Autodesk Fusion 360 part; units mm, degrees
(part 3 of 4)
  line L296 (28.3401, 40.7282) -> (28.1058, 40.494)
  line L297 (25.2342, 40.494) -> (25, 40.7282)
  line L298 (28.1058, 40.494) -> (27.7742, 40.494)
  line L299 (28.1058, 40.494) -> (27.7742, 40.494)
  line L300 (25.8, 40.7282) -> (25.5658, 40.494)
  line L301 (28.3401, 41.0598) -> (28.3401, 40.7282)
  line L302 (25.8, 41.0598) -> (25.8, 40.7282)
  line L303 (25.5658, 41.294) -> (25.8, 41.0598)
  line L304 (25.5658, 40.494) -> (25.2342, 40.494)
  line L305 (25.2342, 41.294) -> (25.5658, 41.294)
  line L306 (25.2342, 41.294) -> (25.5658, 41.294)
  line L307 (25, 40.7282) -> (25, 41.0598)
  line L308 (25, 40.7282) -> (25, 41.0598)
  line L309 (25.8, 41.0598) -> (25.8, 40.7282)
  line L310 (25.5658, 41.294) -> (25.8, 41.0598)
  line L311 (25.8, 40.7282) -> (25.5658, 40.494)
  line L312 (25, 40.7282) -> (25, 41.0598)
  line L313 (25.5658, 40.494) -> (25.2342, 40.494)
  line L314 (25.2342, 45.2311) -> (25.5658, 45.2311)
  line L315 (28.1058, 45.2311) -> (28.3401, 44.9968)
  line L316 (28.1058, 45.2311) -> (28.3401, 44.9968)
  line L317 (28.3401, 44.6652) -> (28.1058, 44.431)
  line L318 (27.54, 44.6652) -> (27.54, 44.9968)
  line L319 (28.1058, 41.294) -> (28.3401, 41.0598)
  line L320 (25, 44.6652) -> (25, 44.9968)
  line L321 (27.7742, 45.2311) -> (28.1058, 45.2311)
  line L322 (28.3401, 44.9968) -> (28.3401, 44.6652)
  line L323 (28.3401, 41.0598) -> (28.3401, 40.7282)
  line L324 (27.54, 44.6652) -> (27.54, 44.9968)
  line L325 (27.54, 44.6652) -> (27.54, 44.9968)
  line L326 (25.8, 44.9968) -> (25.8, 44.6652)
  line L327 (27.54, 41.0598) -> (27.7742, 41.294)
  line L328 (25.5658, 45.2311) -> (25.8, 44.9968)
  line L329 (25.2342, 44.431) -> (25, 44.6652)
  line L330 (25.2342, 44.431) -> (25, 44.6652)
  line L331 (28.1058, 44.431) -> (27.7742, 44.431)
  line L332 (25.5658, 44.431) -> (25.2342, 44.431)
  line L333 (25, 44.6652) -> (25, 44.9968)
  line L334 (27.7742, 41.294) -> (28.1058, 41.294)
  line L335 (25.8, 44.6652) -> (25.5658, 44.431)
  line L336 (27.7742, 44.431) -> (27.54, 44.6652)
  line L337 (27.54, 40.7282) -> (27.54, 41.0598)
  line L338 (25.8, 44.6652) -> (25.5658, 44.431)
  line L339 (25, 44.6652) -> (25, 44.9968)
  line L340 (27.54, 44.9968) -> (27.7742, 45.2311)
  line L341 (28.3401, 44.6652) -> (28.1058, 44.431)
  line L342 (27.7742, 40.494) -> (27.54, 40.7282)
  line L343 (25, 44.9968) -> (25.2342, 45.2311)
  line L344 (10.1791, 41.1868) -> (10.1791, 40.8552)
  line L345 (9.3789, 41.1868) -> (9.6132, 41.4211)
  line L346 (25, 44.6652) -> (25, 44.9968)
  line L347 (12.1532, 40.621) -> (11.919, 40.8552)
  line L348 (9.6132, 41.4211) -> (9.9448, 41.4211)
  line L349 (12.7191, 41.1868) -> (12.7191, 40.8552)
  line L350 (25.5658, 44.431) -> (25.2342, 44.431)
  line L351 (10.1791, 40.8552) -> (9.9448, 40.621)
  line L352 (9.6132, 40.621) -> (9.3789, 40.8552)
  line L353 (27.7742, 45.2311) -> (28.1058, 45.2311)
  line L354 (28.1058, 44.431) -> (27.7742, 44.431)
  line L355 (27.54, 44.9968) -> (27.7742, 45.2311)
  line L356 (27.54, 44.6652) -> (27.54, 44.9968)
  line L357 (28.3401, 44.9968) -> (28.3401, 44.6652)
  line L358 (27.7742, 44.431) -> (27.54, 44.6652)
  line L359 (12.1532, 41.4211) -> (12.4848, 41.4211)
  line L360 (9.3789, 40.8552) -> (9.379, 41.1868)
  line L361 (12.7191, 41.1868) -> (12.7191, 40.8552)
  line L362 (11.919, 41.1868) -> (12.1532, 41.4211)
  line L363 (25.8, 44.9968) -> (25.8, 44.6652)
  line L364 (25.2342, 45.2311) -> (25.5658, 45.2311)
  line L365 (11.919, 40.8552) -> (11.919, 41.1868)
  line L366 (25, 44.9968) -> (25.2342, 45.2311)
  line L367 (12.7191, 40.8552) -> (12.4848, 40.621)
  line L368 (9.9448, 40.621) -> (9.6132, 40.621)
  line L369 (12.7191, 40.8552) -> (12.4848, 40.621)
  line L370 (25.5658, 45.2311) -> (25.8, 44.9968)
  line L371 (12.4848, 41.4211) -> (12.7191, 41.1868)
  arc A1067 (11.811, 48.133) -> (11.811, 48.895) centre (11.811, 48.514) ccw
  line L372 (11.811, 45.974) -> (10.287, 45.974)
  line L373 (10.414, 18.415) -> (8.89, 18.415)
  line L374 (9.6132, 41.4211) -> (9.9448, 41.4211)
  line L375 (17.554, 43.934) -> (16.046, 43.934)
  line L376 (11.811, 48.514) -> (10.287, 48.514)
  line L377 (10.414, 13.335) -> (8.89, 13.335)
  arc A1068 (10.414, 15.494) -> (10.414, 16.256) centre (10.414, 15.875) ccw
  line L378 (11.811, 45.974) -> (10.287, 45.974)
  line L379 (12.4848, 40.621) -> (12.1532, 40.621)
  line L380 (10.1791, 41.1868) -> (10.1791, 40.8552)
  arc A1069 (10.287, 48.895) -> (10.287, 48.133) centre (10.287, 48.514) ccw
  line L381 (11.811, 48.514) -> (10.287, 48.514)
  arc A1070 (10.287, 46.355) -> (10.287, 45.593) centre (10.287, 45.974) ccw
  line L382 (9.6132, 40.621) -> (9.3789, 40.8552)
  arc A1071 (10.287, 46.355) -> (10.287, 45.593) centre (10.287, 45.974) ccw
  line L383 (12.7191, 41.1868) -> (12.7191, 40.8552)
  line L384 (9.3789, 40.8552) -> (9.379, 41.1868)
  line L385 (11.919, 40.8552) -> (11.919, 41.1868)
  line L386 (12.4848, 41.4211) -> (12.7191, 41.1868)
  arc A1072 (11.811, 45.593) -> (11.811, 46.355) centre (11.811, 45.974) ccw
  line L387 (17.554, 42.426) -> (17.554, 43.934)
  line L388 (10.414, 15.875) -> (8.89, 15.875)
  line L389 (9.9448, 40.621) -> (9.6132, 40.621)
  arc A1073 (8.89, 18.796) -> (8.89, 18.034) centre (8.89, 18.415) ccw
  line L390 (9.3789, 41.1868) -> (9.6132, 41.4211)
  arc A1074 (11.811, 48.133) -> (11.811, 48.895) centre (11.811, 48.514) ccw
  line L391 (10.414, 13.335) -> (8.89, 13.335)
  line L392 (12.4848, 40.621) -> (12.1532, 40.621)
  arc A1075 (10.414, 18.034) -> (10.414, 18.796) centre (10.414, 18.415) ccw
  arc A1076 (8.89, 16.256) -> (8.89, 15.494) centre (8.89, 15.875) ccw
  arc A1077 (10.287, 48.895) -> (10.287, 48.133) centre (10.287, 48.514) ccw
  arc A1078 (8.89, 18.796) -> (8.89, 18.034) centre (8.89, 18.415) ccw
  line L393 (10.1791, 41.1868) -> (10.1791, 40.8552)
  line L394 (12.1532, 40.621) -> (11.919, 40.8552)
  line L395 (9.9448, 41.4211) -> (10.1791, 41.1868)
  line L396 (10.1791, 41.1868) -> (10.1791, 40.8552)
  line L397 (10.414, 18.415) -> (8.89, 18.415)
  line L398 (16.046, 42.426) -> (17.554, 42.426)
  line L399 (11.919, 41.1868) -> (12.1532, 41.4211)
  line L400 (12.7191, 41.1868) -> (12.7191, 40.8552)
  line L401 (9.9448, 41.4211) -> (10.1791, 41.1868)
  line L402 (12.1532, 41.4211) -> (12.4848, 41.4211)
  line L403 (10.1791, 40.8552) -> (9.9448, 40.621)
  arc A1079 (11.811, 45.593) -> (11.811, 46.355) centre (11.811, 45.974) ccw
  arc A1080 (10.414, 18.034) -> (10.414, 18.796) centre (10.414, 18.415) ccw
  line L404 (23.7998, 7.7568) -> (23.9932, 7.9502)
  line L405 (24.4602, 15.1032) -> (24.2668, 14.9098)
  line L406 (24.4602, 7.7568) -> (24.4602, 7.4832)
  line L407 (24.4602, 15.1032) -> (24.2668, 14.9098)
  line L408 (23.9932, 14.9098) -> (23.7998, 15.1032)
  line L409 (24.2668, 7.2898) -> (23.9932, 7.2898)
  line L410 (24.2668, 14.9098) -> (23.9932, 14.9098)
  line L411 (24.4602, 7.7568) -> (24.4602, 7.4832)
  line L412 (23.9932, 15.5702) -> (24.2668, 15.5702)
  line L413 (24.2668, 14.9098) -> (23.9932, 14.9098)
  line L414 (24.2668, 15.5702) -> (24.4602, 15.3768)
  line L415 (24.2668, 14.9098) -> (23.9932, 14.9098)
  line L416 (23.9932, 15.5702) -> (24.2668, 15.5702)
  line L417 (24.2668, 7.2898) -> (23.9932, 7.2898)
  arc A1081 (10.414, 15.494) -> (10.414, 16.256) centre (10.414, 15.875) ccw
  arc A1082 (16.423, 48.26) -> (17.177, 48.26) centre (16.8, 48.26) ccw
  line L418 (24.4602, 7.4832) -> (24.2668, 7.2898)
  line L419 (24.2668, 7.2898) -> (23.9932, 7.2898)
  line L420 (23.9932, 14.9098) -> (23.7998, 15.1032)
  line L421 (24.4602, 15.3768) -> (24.4602, 15.1032)
  line L422 (24.2668, 7.2898) -> (23.9932, 7.2898)
  arc A1083 (17.177, 48.26) -> (16.423, 48.26) centre (16.8, 48.26) ccw
  line L423 (24.2668, 7.9502) -> (24.4602, 7.7568)
  line L424 (23.7998, 15.1032) -> (23.7998, 15.3768)
  arc A1084 (10.414, 12.954) -> (10.414, 13.716) centre (10.414, 13.335) ccw
  line L425 (10.414, 15.875) -> (8.89, 15.875)
  line L426 (17.554, 43.934) -> (16.046, 43.934)
  arc A1085 (16.423, 45.72) -> (17.177, 45.72) centre (16.8, 45.72) ccw
  line L427 (16.046, 42.426) -> (17.554, 42.426)
  line L428 (23.9932, 7.9502) -> (24.2668, 7.9502)
  arc A1086 (17.177, 45.72) -> (16.423, 45.72) centre (16.8, 45.72) ccw
  arc A1087 (8.89, 13.716) -> (8.89, 12.954) centre (8.89, 13.335) ccw
  arc A1088 (17.177, 48.26) -> (16.423, 48.26) centre (16.8, 48.26) ccw
  line L429 (24.2668, 15.5702) -> (24.4602, 15.3768)
  line L430 (23.7998, 7.7568) -> (23.9932, 7.9502)
  line L431 (23.7998, 15.3768) -> (23.9932, 15.5702)
  line L432 (16.046, 43.934) -> (16.046, 42.426)
  line L433 (23.7998, 15.1032) -> (23.7998, 15.3768)
  arc A1089 (27.686, 29.21) -> (27.686, 29.972) centre (27.686, 29.591) ccw
  line L434 (27.686, 34.671) -> (26.162, 34.671)
  arc A1090 (8.89, 13.716) -> (8.89, 12.954) centre (8.89, 13.335) ccw
  line L435 (24.4602, 7.4832) -> (24.2668, 7.2898)
  arc A1091 (26.162, 27.432) -> (26.162, 26.67) centre (26.162, 27.051) ccw
  line L436 (24.2668, 14.9098) -> (23.9932, 14.9098)
  line L437 (27.686, 32.131) -> (26.162, 32.131)
  arc A1092 (16.423, 48.26) -> (17.177, 48.26) centre (16.8, 48.26) ccw
  arc A1093 (17.177, 45.72) -> (16.423, 45.72) centre (16.8, 45.72) ccw
  line L438 (24.2668, 7.9502) -> (24.4602, 7.7568)
  line L439 (23.9932, 7.9502) -> (24.2668, 7.9502)
  line L440 (16.046, 43.934) -> (16.046, 42.426)
  line L441 (23.9932, 7.2898) -> (23.7998, 7.4832)
  arc A1094 (16.423, 45.72) -> (17.177, 45.72) centre (16.8, 45.72) ccw
  arc A1095 (8.89, 16.256) -> (8.89, 15.494) centre (8.89, 15.875) ccw
  line L442 (17.554, 42.426) -> (17.554, 43.934)
  line L443 (23.7998, 7.4832) -> (23.7998, 7.7568)
  arc A1096 (10.414, 12.954) -> (10.414, 13.716) centre (10.414, 13.335) ccw
  line L444 (23.7998, 7.4832) -> (23.7998, 7.7568)
  line L445 (23.9932, 7.2898) -> (23.7998, 7.4832)
  line L446 (24.4602, 15.3768) -> (24.4602, 15.1032)
  line L447 (23.7998, 15.3768) -> (23.9932, 15.5702)
  arc A1097 (27.686, 36.83) -> (27.686, 37.592) centre (27.686, 37.211) ccw
  line L448 (27.686, 34.671) -> (26.162, 34.671)
  arc A1098 (26.162, 32.512) -> (26.162, 31.75) centre (26.162, 32.131) ccw
  arc A1099 (27.686, 31.75) -> (27.686, 32.512) centre (27.686, 32.131) ccw
  arc A1100 (27.686, 34.29) -> (27.686, 35.052) centre (27.686, 34.671) ccw
  arc A1101 (27.686, 36.83) -> (27.686, 37.592) centre (27.686, 37.211) ccw
  arc A1102 (26.162, 35.052) -> (26.162, 34.29) centre (26.162, 34.671) ccw
  line L449 (27.686, 37.211) -> (26.162, 37.211)
  line L450 (27.686, 29.591) -> (26.162, 29.591)
  arc A1103 (26.162, 29.972) -> (26.162, 29.21) centre (26.162, 29.591) ccw
  line L451 (27.686, 19.431) -> (26.162, 19.431)
  line L452 (27.686, 27.051) -> (26.162, 27.051)
  arc A1104 (27.686, 26.67) -> (27.686, 27.432) centre (27.686, 27.051) ccw
  arc A1105 (26.162, 24.892) -> (26.162, 24.13) centre (26.162, 24.511) ccw
  arc A1106 (27.686, 24.13) -> (27.686, 24.892) centre (27.686, 24.511) ccw
  line L453 (27.686, 19.431) -> (26.162, 19.431)
  arc A1107 (26.162, 19.812) -> (26.162, 19.05) centre (26.162, 19.431) ccw
  line L454 (27.686, 21.971) -> (26.162, 21.971)
  arc A1108 (27.686, 34.29) -> (27.686, 35.052) centre (27.686, 34.671) ccw
  line L455 (27.686, 24.511) -> (26.162, 24.511)
  arc A1109 (26.162, 22.352) -> (26.162, 21.59) centre (26.162, 21.971) ccw
  arc A1110 (27.686, 24.13) -> (27.686, 24.892) centre (27.686, 24.511) ccw
  arc A1111 (26.162, 27.432) -> (26.162, 26.67) centre (26.162, 27.051) ccw
  arc A1112 (27.686, 19.05) -> (27.686, 19.812) centre (27.686, 19.431) ccw
  arc A1113 (27.686, 26.67) -> (27.686, 27.432) centre (27.686, 27.051) ccw
  arc A1114 (26.162, 22.352) -> (26.162, 21.59) centre (26.162, 21.971) ccw
  line L456 (27.686, 21.971) -> (26.162, 21.971)
  line L457 (27.686, 29.591) -> (26.162, 29.591)
  line L458 (27.686, 27.051) -> (26.162, 27.051)
  line L459 (27.686, 32.131) -> (26.162, 32.131)
  line L460 (27.686, 24.511) -> (26.162, 24.511)
  arc A1115 (27.686, 21.59) -> (27.686, 22.352) centre (27.686, 21.971) ccw
  arc A1116 (27.686, 29.21) -> (27.686, 29.972) centre (27.686, 29.591) ccw
  arc A1117 (26.162, 37.592) -> (26.162, 36.83) centre (26.162, 37.211) ccw
  arc A1118 (26.162, 35.052) -> (26.162, 34.29) centre (26.162, 34.671) ccw
  line L461 (27.686, 37.211) -> (26.162, 37.211)
  arc A1119 (27.686, 21.59) -> (27.686, 22.352) centre (27.686, 21.971) ccw
  arc A1120 (26.162, 32.512) -> (26.162, 31.75) centre (26.162, 32.131) ccw
  arc A1121 (13.462, 19.812) -> (13.462, 19.05) centre (13.462, 19.431) ccw
  arc A1122 (13.462, 32.512) -> (13.462, 31.75) centre (13.462, 32.131) ccw
  arc A1123 (13.462, 22.352) -> (13.462, 21.59) centre (13.462, 21.971) ccw
  arc A1124 (27.686, 19.05) -> (27.686, 19.812) centre (27.686, 19.431) ccw
  arc A1125 (26.162, 24.892) -> (26.162, 24.13) centre (26.162, 24.511) ccw
  arc A1126 (26.162, 37.592) -> (26.162, 36.83) centre (26.162, 37.211) ccw
  arc A1127 (27.686, 31.75) -> (27.686, 32.512) centre (27.686, 32.131) ccw
  line L462 (13.462, 24.511) -> (14.986, 24.511)
  arc A1128 (13.462, 22.352) -> (13.462, 21.59) centre (13.462, 21.971) ccw
  arc A1129 (13.462, 24.892) -> (13.462, 24.13) centre (13.462, 24.511) ccw
  arc A1130 (14.986, 29.21) -> (14.986, 29.972) centre (14.986, 29.591) ccw
  line L463 (13.462, 19.431) -> (14.986, 19.431)
  arc A1131 (14.986, 19.05) -> (14.986, 19.812) centre (14.986, 19.431) ccw
  arc A1132 (26.162, 19.812) -> (26.162, 19.05) centre (26.162, 19.431) ccw
  line L464 (13.462, 24.511) -> (14.986, 24.511)
  arc A1133 (13.462, 29.972) -> (13.462, 29.21) centre (13.462, 29.591) ccw
  arc A1134 (26.162, 29.972) -> (26.162, 29.21) centre (26.162, 29.591) ccw
  arc A1135 (14.986, 19.05) -> (14.986, 19.812) centre (14.986, 19.431) ccw
  line L465 (13.462, 21.971) -> (14.986, 21.971)
  arc A1136 (14.986, 31.75) -> (14.986, 32.512) centre (14.986, 32.131) ccw
  arc A1137 (14.986, 29.21) -> (14.986, 29.972) centre (14.986, 29.591) ccw
  arc A1138 (13.462, 27.432) -> (13.462, 26.67) centre (13.462, 27.051) ccw
  line L466 (13.462, 29.591) -> (14.986, 29.591)
  line L467 (13.462, 32.131) -> (14.986, 32.131)
  line L468 (13.462, 37.211) -> (14.986, 37.211)
  line L469 (13.462, 27.051) -> (14.986, 27.051)
  arc A1139 (14.986, 26.67) -> (14.986, 27.432) centre (14.986, 27.051) ccw
  arc A1140 (14.986, 21.59) -> (14.986, 22.352) centre (14.986, 21.971) ccw
  arc A1141 (14.986, 24.13) -> (14.986, 24.892) centre (14.986, 24.511) ccw
  arc A1142 (13.462, 32.512) -> (13.462, 31.75) centre (13.462, 32.131) ccw
  arc A1143 (13.462, 29.972) -> (13.462, 29.21) centre (13.462, 29.591) ccw
  line L470 (13.462, 34.671) -> (14.986, 34.671)
  line L471 (13.462, 29.591) -> (14.986, 29.591)
  arc A1144 (13.462, 35.052) -> (13.462, 34.29) centre (13.462, 34.671) ccw
  line L472 (13.462, 32.131) -> (14.986, 32.131)
  arc A1145 (13.462, 35.052) -> (13.462, 34.29) centre (13.462, 34.671) ccw
  line L473 (13.462, 34.671) -> (14.986, 34.671)
  arc A1146 (14.986, 34.29) -> (14.986, 35.052) centre (14.986, 34.671) ccw
  arc A1147 (13.462, 27.432) -> (13.462, 26.67) centre (13.462, 27.051) ccw
  arc A1148 (14.986, 34.29) -> (14.986, 35.052) centre (14.986, 34.671) ccw
  line L474 (13.462, 21.971) -> (14.986, 21.971)
  arc A1149 (30.8896, 34.935) -> (29.9244, 34.935) centre (30.407, 34.935) ccw
  line L475 (13.462, 37.211) -> (14.986, 37.211)
  arc A1150 (14.986, 36.83) -> (14.986, 37.592) centre (14.986, 37.211) ccw
  arc A1151 (5.4846, 24.775) -> (4.5194, 24.775) centre (5.002, 24.775) ccw
  arc A1152 (4.5194, 34.935) -> (5.4846, 34.935) centre (5.002, 34.935) ccw
  arc A1153 (4.5194, 42.555) -> (5.4846, 42.555) centre (5.002, 42.555) ccw
  arc A1154 (14.986, 36.83) -> (14.986, 37.592) centre (14.986, 37.211) ccw
  arc A1155 (13.462, 37.592) -> (13.462, 36.83) centre (13.462, 37.211) ccw
  arc A1156 (14.986, 26.67) -> (14.986, 27.432) centre (14.986, 27.051) ccw
  arc A1157 (5.4846, 14.615) -> (4.5194, 14.615) centre (5.002, 14.615) ccw
  arc A1158 (4.5194, 42.555) -> (5.4846, 42.555) centre (5.002, 42.555) ccw
  arc A1159 (4.5194, 24.775) -> (5.4846, 24.775) centre (5.002, 24.775) ccw
  arc A1160 (5.4846, 42.555) -> (4.5194, 42.555) centre (5.002, 42.555) ccw
  arc A1161 (4.5194, 14.615) -> (5.4846, 14.615) centre (5.002, 14.615) ccw
  arc A1162 (13.462, 24.892) -> (13.462, 24.13) centre (13.462, 24.511) ccw
  line L476 (13.462, 19.431) -> (14.986, 19.431)
  arc A1163 (14.986, 31.75) -> (14.986, 32.512) centre (14.986, 32.131) ccw
  arc A1164 (14.986, 21.59) -> (14.986, 22.352) centre (14.986, 21.971) ccw
  arc A1165 (29.9244, 34.935) -> (30.8896, 34.935) centre (30.407, 34.935) ccw
  arc A1166 (14.986, 24.13) -> (14.986, 24.892) centre (14.986, 24.511) ccw
  line L477 (13.462, 27.051) -> (14.986, 27.051)
  arc A1167 (13.462, 19.812) -> (13.462, 19.05) centre (13.462, 19.431) ccw
  arc A1168 (13.462, 37.592) -> (13.462, 36.83) centre (13.462, 37.211) ccw
  arc A1169 (4.5194, 12.075) -> (5.4846, 12.075) centre (5.002, 12.075) ccw
  arc A1170 (5.4846, 34.935) -> (4.5194, 34.935) centre (5.002, 34.935) ccw
  arc A1171 (5.4846, 14.615) -> (4.5194, 14.615) centre (5.002, 14.615) ccw
  arc A1172 (4.5194, 32.395) -> (5.4846, 32.395) centre (5.002, 32.395) ccw
  arc A1173 (5.4846, 34.935) -> (4.5194, 34.935) centre (5.002, 34.935) ccw
  arc A1174 (4.5194, 32.395) -> (5.4846, 32.395) centre (5.002, 32.395) ccw
  arc A1175 (5.4846, 32.395) -> (4.5194, 32.395) centre (5.002, 32.395) ccw
  arc A1176 (5.4846, 24.775) -> (4.5194, 24.775) centre (5.002, 24.775) ccw
  arc A1177 (5.4846, 12.075) -> (4.5194, 12.075) centre (5.002, 12.075) ccw
  arc A1178 (4.5194, 12.075) -> (5.4846, 12.075) centre (5.002, 12.075) ccw
  arc A1179 (4.5194, 14.615) -> (5.4846, 14.615) centre (5.002, 14.615) ccw
  arc A1180 (5.4846, 32.395) -> (4.5194, 32.395) centre (5.002, 32.395) ccw
  arc A1181 (5.4846, 12.075) -> (4.5194, 12.075) centre (5.002, 12.075) ccw
  arc A1182 (4.5194, 34.935) -> (5.4846, 34.935) centre (5.002, 34.935) ccw
  arc A1183 (5.4846, 42.555) -> (4.5194, 42.555) centre (5.002, 42.555) ccw
  arc A1184 (4.5194, 19.695) -> (5.4846, 19.695) centre (5.002, 19.695) ccw
  arc A1185 (29.9244, 32.395) -> (30.8896, 32.395) centre (30.407, 32.395) ccw
  arc A1186 (29.9244, 24.775) -> (30.8896, 24.775) centre (30.407, 24.775) ccw
  arc A1187 (29.9244, 34.935) -> (30.8896, 34.935) centre (30.407, 34.935) ccw
  arc A1188 (5.4846, 22.235) -> (4.5194, 22.235) centre (5.002, 22.235) ccw
  arc A1189 (4.5194, 19.695) -> (5.4846, 19.695) centre (5.002, 19.695) ccw
  arc A1190 (30.8896, 32.395) -> (29.9244, 32.395) centre (30.407, 32.395) ccw
  arc A1191 (5.4846, 27.315) -> (4.5194, 27.315) centre (5.002, 27.315) ccw
  arc A1192 (4.5194, 22.235) -> (5.4846, 22.235) centre (5.002, 22.235) ccw
  arc A1193 (30.8896, 27.315) -> (29.9244, 27.315) centre (30.407, 27.315) ccw
  arc A1194 (5.4846, 37.475) -> (4.5194, 37.475) centre (5.002, 37.475) ccw
  arc A1195 (4.5194, 27.315) -> (5.4846, 27.315) centre (5.002, 27.315) ccw
  arc A1196 (30.8896, 19.695) -> (29.9244, 19.695) centre (30.407, 19.695) ccw
  arc A1197 (4.5194, 24.775) -> (5.4846, 24.775) centre (5.002, 24.775) ccw
  arc A1198 (4.5194, 22.235) -> (5.4846, 22.235) centre (5.002, 22.235) ccw
  arc A1199 (4.5194, 17.155) -> (5.4846, 17.155) centre (5.002, 17.155) ccw
  arc A1200 (5.4846, 17.155) -> (4.5194, 17.155) centre (5.002, 17.155) ccw
  arc A1201 (30.8896, 34.935) -> (29.9244, 34.935) centre (30.407, 34.935) ccw
  arc A1202 (5.4846, 19.695) -> (4.5194, 19.695) centre (5.002, 19.695) ccw
  arc A1203 (29.9244, 22.235) -> (30.8896, 22.235) centre (30.407, 22.235) ccw
  arc A1204 (30.8896, 14.615) -> (29.9244, 14.615) centre (30.407, 14.615) ccw
  arc A1205 (5.4846, 37.475) -> (4.5194, 37.475) centre (5.002, 37.475) ccw
  arc A1206 (30.8896, 37.475) -> (29.9244, 37.475) centre (30.407, 37.475) ccw
  arc A1207 (29.9244, 37.475) -> (30.8896, 37.475) centre (30.407, 37.475) ccw
  arc A1208 (5.4846, 6.995) -> (4.5194, 6.995) centre (5.002, 6.995) ccw
  arc A1209 (29.9244, 29.855) -> (30.8896, 29.855) centre (30.407, 29.855) ccw
  arc A1210 (4.5194, 9.535) -> (5.4846, 9.535) centre (5.002, 9.535) ccw
  arc A1211 (5.4846, 9.535) -> (4.5194, 9.535) centre (5.002, 9.535) ccw
  arc A1212 (30.8896, 22.235) -> (29.9244, 22.235) centre (30.407, 22.235) ccw
  arc A1213 (29.9244, 14.615) -> (30.8896, 14.615) centre (30.407, 14.615) ccw
  arc A1214 (29.9244, 24.775) -> (30.8896, 24.775) centre (30.407, 24.775) ccw
  arc A1215 (5.4846, 9.535) -> (4.5194, 9.535) centre (5.002, 9.535) ccw
  arc A1216 (30.8896, 24.775) -> (29.9244, 24.775) centre (30.407, 24.775) ccw
  arc A1217 (5.4846, 19.695) -> (4.5194, 19.695) centre (5.002, 19.695) ccw
  arc A1218 (5.4846, 17.155) -> (4.5194, 17.155) centre (5.002, 17.155) ccw
  arc A1219 (29.9244, 27.315) -> (30.8896, 27.315) centre (30.407, 27.315) ccw
  arc A1220 (30.8896, 37.475) -> (29.9244, 37.475) centre (30.407, 37.475) ccw
  arc A1221 (29.9244, 29.855) -> (30.8896, 29.855) centre (30.407, 29.855) ccw
  arc A1222 (4.5194, 9.535) -> (5.4846, 9.535) centre (5.002, 9.535) ccw
  arc A1223 (4.5194, 6.995) -> (5.4846, 6.995) centre (5.002, 6.995) ccw
  arc A1224 (30.8896, 24.775) -> (29.9244, 24.775) centre (30.407, 24.775) ccw
  arc A1225 (5.4846, 27.315) -> (4.5194, 27.315) centre (5.002, 27.315) ccw
  arc A1226 (5.4846, 6.995) -> (4.5194, 6.995) centre (5.002, 6.995) ccw
  arc A1227 (30.8896, 29.855) -> (29.9244, 29.855) centre (30.407, 29.855) ccw
  arc A1228 (4.5194, 27.315) -> (5.4846, 27.315) centre (5.002, 27.315) ccw
  arc A1229 (29.9244, 32.395) -> (30.8896, 32.395) centre (30.407, 32.395) ccw
  arc A1230 (5.4846, 22.235) -> (4.5194, 22.235) centre (5.002, 22.235) ccw
  arc A1231 (4.5194, 6.995) -> (5.4846, 6.995) centre (5.002, 6.995) ccw
  arc A1232 (4.5194, 37.475) -> (5.4846, 37.475) centre (5.002, 37.475) ccw
  arc A1233 (4.5194, 17.155) -> (5.4846, 17.155) centre (5.002, 17.155) ccw
  arc A1234 (5.4846, 29.855) -> (4.5194, 29.855) centre (5.002, 29.855) ccw
  arc A1235 (5.4846, 29.855) -> (4.5194, 29.855) centre (5.002, 29.855) ccw
  arc A1236 (30.8896, 32.395) -> (29.9244, 32.395) centre (30.407, 32.395) ccw
  arc A1237 (23.55, 51.7075) -> (23.55, 51.7325) centre (23.55, 51.72) ccw
  line L478 (23.55, 51.72) -> (23.55, 39.62)
  arc A1238 (23.5625, 51.72) -> (23.5375, 51.72) centre (23.55, 51.72) ccw
  arc A1239 (23.55, 39.6075) -> (23.55, 39.6325) centre (23.55, 39.62) ccw
  arc A1240 (14.55, 39.6325) -> (14.55, 39.6075) centre (14.55, 39.62) ccw
  line L479 (14.55, 51.72) -> (23.55, 51.72)
  arc A1241 (14.5375, 39.62) -> (14.5625, 39.62) centre (14.55, 39.62) ccw
  arc A1242 (14.55, 51.7325) -> (14.55, 51.7075) centre (14.55, 51.72) ccw
  line L480 (14.55, 39.62) -> (14.55, 51.72)
  arc A1243 (23.5375, 39.62) -> (23.5625, 39.62) centre (23.55, 39.62) ccw
  line L481 (23.55, 39.62) -> (14.55, 39.62)
  arc A1244 (14.5625, 51.72) -> (14.5375, 51.72) centre (14.55, 51.72) ccw
  line L482 (6.3786, 40.894) -> (9.779, 41.021)
sketch "Universal_Board_Side_Mount (1)" plane through (0, 0, 0) normal (0, 0, 1) x (1, 0, 0)
  line L0 (25.5658, 41.294) -> (25.8001, 41.0598)
  line L1 (28.1058, 41.294) -> (28.3401, 41.0598)
  line L2 (25.8001, 41.0598) -> (25.8, 40.7282)
  line L3 (25, 40.7282) -> (25, 41.0598)
  line L4 (27.7742, 40.494) -> (27.54, 40.7282)
  line L5 (27.54, 40.7282) -> (27.54, 41.0598)
  line L6 (25, 40.7282) -> (25, 41.0598)
  line L7 (25.5658, 40.494) -> (25.2342, 40.494)
  line L8 (27.54, 41.0598) -> (27.7742, 41.294)
  line L9 (27.7742, 41.294) -> (28.1058, 41.294)
  line L10 (25.2342, 41.294) -> (25.5658, 41.294)
  line L11 (27.54, 40.7282) -> (27.54, 41.0598)
  line L12 (27.54, 40.7282) -> (27.54, 41.0598)
  line L13 (28.3401, 41.0598) -> (28.3401, 40.7282)
  line L14 (25, 40.7282) -> (25, 41.0598)
  line L15 (27.54, 41.0598) -> (27.7742, 41.294)
  line L16 (25.8, 40.7282) -> (25.5658, 40.494)
  line L17 (27.54, 40.7282) -> (27.54, 41.0598)
  line L18 (25.8001, 41.0598) -> (25.8, 40.7282)
  line L19 (25.2342, 40.494) -> (25, 40.7282)
  line L20 (28.3401, 40.7282) -> (28.1058, 40.494)
  line L21 (25.2342, 41.294) -> (25.5658, 41.294)
  line L22 (25, 40.7282) -> (25, 41.0598)
  line L23 (25.5658, 41.294) -> (25.8001, 41.0598)
  line L24 (25.8, 40.7282) -> (25.5658, 40.494)
  line L25 (27.7742, 41.294) -> (28.1058, 41.294)
  line L26 (25.5658, 40.494) -> (25.2342, 40.494)
  line L27 (25.2342, 40.494) -> (25, 40.7282)
  line L28 (28.1058, 41.294) -> (28.3401, 41.0598)
  line L29 (25, 41.0598) -> (25.2342, 41.294)
  line L30 (28.3401, 41.0598) -> (28.3401, 40.7282)
  line L31 (28.1058, 40.494) -> (27.7742, 40.494)
  line L32 (27.7742, 40.494) -> (27.54, 40.7282)
  line L33 (28.1058, 40.494) -> (27.7742, 40.494)
  line L34 (27.54, 44.9968) -> (27.7742, 45.2311)
  line L35 (28.3401, 40.7282) -> (28.1058, 40.494)
  line L36 (25, 41.0598) -> (25.2342, 41.294)
  line L37 (25.2342, 45.2311) -> (25.5658, 45.2311)
  line L38 (25.8, 44.9968) -> (25.8, 44.6652)
  line L39 (25.5658, 44.431) -> (25.2342, 44.431)
  line L40 (27.7742, 45.2311) -> (28.1058, 45.2311)
  line L41 (27.7742, 45.2311) -> (28.1058, 45.2311)
  line L42 (25, 44.6652) -> (25, 44.9968)
  line L43 (25.2342, 44.431) -> (25, 44.6652)
  line L44 (25.5658, 44.431) -> (25.2342, 44.431)
  line L45 (25, 44.9968) -> (25.2342, 45.2311)
  line L46 (25, 44.6652) -> (25, 44.9968)
  line L47 (28.3401, 44.6652) -> (28.1058, 44.431)
  line L48 (28.3401, 44.9968) -> (28.3401, 44.6652)
  line L49 (27.7742, 44.431) -> (27.54, 44.6652)
  line L50 (25.2342, 44.431) -> (25, 44.6652)
  line L51 (27.54, 44.9968) -> (27.7742, 45.2311)
  line L52 (25, 44.6652) -> (25, 44.9968)
  line L53 (27.54, 44.6652) -> (27.54, 44.9968)
  line L54 (28.1058, 44.431) -> (27.7742, 44.431)
  line L55 (25.8, 44.9968) -> (25.8, 44.6652)
  line L56 (25.8, 44.6652) -> (25.5658, 44.431)
  line L57 (28.1058, 45.2311) -> (28.3401, 44.9968)
  line L58 (25.8, 44.6652) -> (25.5658, 44.431)
  line L59 (25, 44.9968) -> (25.2342, 45.2311)
  arc A0 (10.414, 18.034) -> (10.414, 18.796) centre (10.414, 18.415) ccw
  line L60 (12.7191, 40.8552) -> (12.4848, 40.621)
  line L61 (12.4848, 40.621) -> (12.1532, 40.621)
  line L62 (12.7191, 41.1868) -> (12.7191, 40.8552)
  line L63 (28.1058, 45.2311) -> (28.3401, 44.9968)
  line L64 (9.3789, 41.1868) -> (9.6132, 41.4211)
  line L65 (12.4848, 41.4211) -> (12.7191, 41.1868)
  line L66 (12.1532, 41.4211) -> (12.4848, 41.4211)
  line L67 (10.1791, 41.1868) -> (10.1791, 40.8552)
  line L68 (25.5658, 45.2311) -> (25.8, 44.9968)
  line L69 (9.6132, 40.621) -> (9.3789, 40.8552)
  line L70 (25.5658, 45.2311) -> (25.8, 44.9968)
  line L71 (12.4848, 41.4211) -> (12.7191, 41.1868)
  line L72 (9.9448, 40.621) -> (9.6132, 40.621)
  line L73 (9.9448, 41.4211) -> (10.1791, 41.1868)
  line L74 (9.9448, 40.621) -> (9.6132, 40.621)
  line L75 (9.6132, 41.4211) -> (9.9448, 41.4211)
  line L76 (25.2342, 45.2311) -> (25.5658, 45.2311)
  line L77 (12.7191, 41.1868) -> (12.7191, 40.8552)
  line L78 (9.9448, 41.4211) -> (10.1791, 41.1868)
  line L79 (12.1532, 40.621) -> (11.919, 40.8552)
  line L80 (11.919, 41.1868) -> (12.1532, 41.4211)
  line L81 (12.7191, 41.1868) -> (12.7191, 40.8552)
  line L82 (11.919, 41.1868) -> (12.1532, 41.4211)
  line L83 (9.3789, 40.8552) -> (9.379, 41.1868)
  arc A1 (10.287, 48.895) -> (10.287, 48.133) centre (10.287, 48.514) ccw
  line L84 (11.811, 48.514) -> (10.287, 48.514)
  line L85 (17.554, 42.426) -> (17.554, 43.934)
  line L86 (17.554, 43.934) -> (16.046, 43.934)
  arc A2 (10.287, 46.355) -> (10.287, 45.593) centre (10.287, 45.974) ccw
  line L87 (11.919, 40.8552) -> (11.919, 41.1868)
  arc A3 (10.287, 48.895) -> (10.287, 48.133) centre (10.287, 48.514) ccw
  arc A4 (10.287, 46.355) -> (10.287, 45.593) centre (10.287, 45.974) ccw
  line L88 (12.7191, 40.8552) -> (12.4848, 40.621)
  line L89 (9.6132, 40.621) -> (9.3789, 40.8552)
  arc A5 (8.89, 16.256) -> (8.89, 15.494) centre (8.89, 15.875) ccw
  line L90 (25, 44.6652) -> (25, 44.9968)
  line L91 (28.3401, 44.6652) -> (28.1058, 44.431)
  line L92 (12.4848, 40.621) -> (12.1532, 40.621)
  line L93 (12.1532, 40.621) -> (11.919, 40.8552)
  line L94 (10.1791, 40.8552) -> (9.9448, 40.621)
  line L95 (11.919, 40.8552) -> (11.919, 41.1868)
  line L96 (12.7191, 41.1868) -> (12.7191, 40.8552)
  line L97 (9.3789, 40.8552) -> (9.379, 41.1868)
  arc A6 (11.811, 48.133) -> (11.811, 48.895) centre (11.811, 48.514) ccw
  line L98 (10.1791, 41.1868) -> (10.1791, 40.8552)
  line L99 (11.811, 45.974) -> (10.287, 45.974)
  line L100 (9.6132, 41.4211) -> (9.9448, 41.4211)
  line L101 (28.3401, 44.9968) -> (28.3401, 44.6652)
  line L102 (11.811, 45.974) -> (10.287, 45.974)
  line L103 (27.54, 44.6652) -> (27.54, 44.9968)
  line L104 (10.1791, 41.1868) -> (10.1791, 40.8552)
  line L105 (12.1532, 41.4211) -> (12.4848, 41.4211)
  line L106 (27.7742, 44.431) -> (27.54, 44.6652)
  line L107 (27.54, 44.6652) -> (27.54, 44.9968)
  line L108 (9.3789, 41.1868) -> (9.6132, 41.4211)
  line L109 (28.1058, 44.431) -> (27.7742, 44.431)
  line L110 (11.811, 48.514) -> (10.287, 48.514)
  arc A7 (11.811, 48.133) -> (11.811, 48.895) centre (11.811, 48.514) ccw
  line L111 (27.54, 44.6652) -> (27.54, 44.9968)
  line L112 (10.1791, 41.1868) -> (10.1791, 40.8552)
  arc A8 (11.811, 45.593) -> (11.811, 46.355) centre (11.811, 45.974) ccw
  line L113 (10.1791, 40.8552) -> (9.9448, 40.621)
  arc A9 (11.811, 45.593) -> (11.811, 46.355) centre (11.811, 45.974) ccw
  arc A10 (17.177, 45.72) -> (16.423, 45.72) centre (16.8, 45.72) ccw
  line L114 (16.046, 43.934) -> (16.046, 42.426)
  arc A11 (10.414, 15.494) -> (10.414, 16.256) centre (10.414, 15.875) ccw
  line L115 (23.7998, 15.1032) -> (23.7998, 15.3768)
  line L116 (24.2668, 14.9098) -> (23.9932, 14.9098)
  line L117 (16.046, 43.934) -> (16.046, 42.426)
  line L118 (24.2668, 7.2898) -> (23.9932, 7.2898)
  line L119 (23.9932, 7.2898) -> (23.7998, 7.4832)
  line L120 (23.9932, 15.5702) -> (24.2668, 15.5702)
  arc A12 (8.89, 18.796) -> (8.89, 18.034) centre (8.89, 18.415) ccw
  arc A13 (8.89, 13.716) -> (8.89, 12.954) centre (8.89, 13.335) ccw
  arc A14 (16.423, 48.26) -> (17.177, 48.26) centre (16.8, 48.26) ccw
  arc A15 (10.414, 18.034) -> (10.414, 18.796) centre (10.414, 18.415) ccw
  line L121 (24.2668, 7.9502) -> (24.4602, 7.7568)
  line L122 (10.414, 18.415) -> (8.89, 18.415)
  arc A16 (10.414, 12.954) -> (10.414, 13.716) centre (10.414, 13.335) ccw
  arc A17 (10.414, 15.494) -> (10.414, 16.256) centre (10.414, 15.875) ccw
  line L123 (16.046, 42.426) -> (17.554, 42.426)
  line L124 (10.414, 13.335) -> (8.89, 13.335)
  line L125 (10.414, 15.875) -> (8.89, 15.875)
  line L126 (17.554, 43.934) -> (16.046, 43.934)
  arc A18 (16.423, 45.72) -> (17.177, 45.72) centre (16.8, 45.72) ccw
  arc A19 (8.89, 18.796) -> (8.89, 18.034) centre (8.89, 18.415) ccw
  line L127 (10.414, 15.875) -> (8.89, 15.875)
  arc A20 (17.177, 48.26) -> (16.423, 48.26) centre (16.8, 48.26) ccw
  arc A21 (8.89, 16.256) -> (8.89, 15.494) centre (8.89, 15.875) ccw
  arc A22 (16.423, 48.26) -> (17.177, 48.26) centre (16.8, 48.26) ccw
  arc A23 (16.423, 45.72) -> (17.177, 45.72) centre (16.8, 45.72) ccw
  arc A24 (17.177, 45.72) -> (16.423, 45.72) centre (16.8, 45.72) ccw
  arc A25 (17.177, 48.26) -> (16.423, 48.26) centre (16.8, 48.26) ccw
  arc A26 (10.414, 12.954) -> (10.414, 13.716) centre (10.414, 13.335) ccw
  line L128 (24.2668, 7.2898) -> (23.9932, 7.2898)
  line L129 (16.046, 42.426) -> (17.554, 42.426)
  line L130 (23.7998, 7.4832) -> (23.7998, 7.7568)
  arc A27 (8.89, 13.716) -> (8.89, 12.954) centre (8.89, 13.335) ccw
  line L131 (10.414, 13.335) -> (8.89, 13.335)
  line L132 (17.554, 42.426) -> (17.554, 43.934)
  line L133 (24.2668, 15.5702) -> (24.4602, 15.3768)
  line L134 (10.414, 18.415) -> (8.89, 18.415)
  line L135 (23.9932, 7.9502) -> (24.2668, 7.9502)
  line L136 (23.9932, 14.9098) -> (23.7998, 15.1032)
  line L137 (24.4602, 15.1032) -> (24.2668, 14.9098)
  line L138 (24.4602, 7.4832) -> (24.2668, 7.2898)
  line L139 (24.2668, 7.2898) -> (23.9932, 7.2898)
  line L140 (23.7998, 7.7568) -> (23.9932, 7.9502)
  line L141 (23.9932, 14.9098) -> (23.7998, 15.1032)
  line L142 (24.4602, 7.4832) -> (24.2668, 7.2898)
  line L143 (23.9932, 7.9502) -> (24.2668, 7.9502)
  line L144 (23.9932, 7.2898) -> (23.7998, 7.4832)
  line L145 (24.4602, 7.7568) -> (24.4602, 7.4832)
  line L146 (24.2668, 15.5702) -> (24.4602, 15.3768)
  line L147 (24.4602, 7.7568) -> (24.4602, 7.4832)
  line L148 (23.7998, 15.3768) -> (23.9932, 15.5702)
  line L149 (24.4602, 15.3768) -> (24.4602, 15.1032)
  line L150 (23.9932, 15.5702) -> (24.2668, 15.5702)
  line L151 (10.541, 28.194) -> (9.017, 28.194)
  line L152 (24.2668, 14.9098) -> (23.9932, 14.9098)
  line L153 (23.7998, 7.4832) -> (23.7998, 7.7568)
  line L154 (24.2668, 14.9098) -> (23.9932, 14.9098)
  line L155 (23.7998, 15.1032) -> (23.7998, 15.3768)
  line L156 (24.4602, 15.3768) -> (24.4602, 15.1032)
  line L157 (23.7998, 15.3768) -> (23.9932, 15.5702)
  line L158 (24.2668, 7.2898) -> (23.9932, 7.2898)
  line L159 (24.4602, 15.1032) -> (24.2668, 14.9098)
  line L160 (24.2668, 7.9502) -> (24.4602, 7.7568)
  arc A28 (10.541, 32.893) -> (10.541, 33.655) centre (10.541, 33.274) ccw
  line L161 (10.541, 25.654) -> (9.017, 25.654)
  line L162 (23.7998, 7.7568) -> (23.9932, 7.9502)
  line L163 (24.2668, 14.9098) -> (23.9932, 14.9098)
  line L164 (27.686, 37.211) -> (26.162, 37.211)
  arc A29 (9.017, 31.115) -> (9.017, 30.353) centre (9.017, 30.734) ccw
  arc A30 (10.541, 27.813) -> (10.541, 28.575) centre (10.541, 28.194) ccw
  arc A31 (27.686, 24.13) -> (27.686, 24.892) centre (27.686, 24.511) ccw
  line L165 (27.686, 34.671) -> (26.162, 34.671)
  arc A32 (27.686, 31.75) -> (27.686, 32.512) centre (27.686, 32.131) ccw
  line L166 (10.541, 33.274) -> (9.017, 33.274)
  arc A33 (10.541, 25.273) -> (10.541, 26.035) centre (10.541, 25.654) ccw
  line L167 (27.686, 21.971) -> (26.162, 21.971)
  arc A34 (27.686, 36.83) -> (27.686, 37.592) centre (27.686, 37.211) ccw
  arc A35 (26.162, 29.972) -> (26.162, 29.21) centre (26.162, 29.591) ccw
  line L168 (27.686, 29.591) -> (26.162, 29.591)
  line L169 (27.686, 27.051) -> (26.162, 27.051)
  arc A36 (26.162, 19.812) -> (26.162, 19.05) centre (26.162, 19.431) ccw
  arc A37 (27.686, 21.59) -> (27.686, 22.352) centre (27.686, 21.971) ccw
  arc A38 (27.686, 26.67) -> (27.686, 27.432) centre (27.686, 27.051) ccw
  arc A39 (26.162, 32.512) -> (26.162, 31.75) centre (26.162, 32.131) ccw
  arc A40 (27.686, 26.67) -> (27.686, 27.432) centre (27.686, 27.051) ccw
  arc A41 (10.541, 30.353) -> (10.541, 31.115) centre (10.541, 30.734) ccw
  arc A42 (10.541, 25.273) -> (10.541, 26.035) centre (10.541, 25.654) ccw
  arc A43 (26.162, 24.892) -> (26.162, 24.13) centre (26.162, 24.511) ccw
  line L170 (10.541, 30.734) -> (9.017, 30.734)
  line L171 (10.541, 33.274) -> (9.017, 33.274)
  line L172 (10.541, 25.654) -> (9.017, 25.654)
  arc A44 (26.162, 27.432) -> (26.162, 26.67) centre (26.162, 27.051) ccw
  arc A45 (27.686, 29.21) -> (27.686, 29.972) centre (27.686, 29.591) ccw
  line L173 (27.686, 32.131) -> (26.162, 32.131)
  arc A46 (27.686, 36.83) -> (27.686, 37.592) centre (27.686, 37.211) ccw
  arc A47 (27.686, 34.29) -> (27.686, 35.052) centre (27.686, 34.671) ccw
  line L174 (27.686, 37.211) -> (26.162, 37.211)
  arc A48 (26.162, 37.592) -> (26.162, 36.83) centre (26.162, 37.211) ccw
  arc A49 (10.541, 30.353) -> (10.541, 31.115) centre (10.541, 30.734) ccw
  arc A50 (9.017, 33.655) -> (9.017, 32.893) centre (9.017, 33.274) ccw
  line L175 (27.686, 24.511) -> (26.162, 24.511)
  arc A51 (27.686, 19.05) -> (27.686, 19.812) centre (27.686, 19.431) ccw
  line L176 (27.686, 29.591) -> (26.162, 29.591)
  arc A52 (27.686, 31.75) -> (27.686, 32.512) centre (27.686, 32.131) ccw
  arc A53 (26.162, 35.052) -> (26.162, 34.29) centre (26.162, 34.671) ccw
  arc A54 (26.162, 22.352) -> (26.162, 21.59) centre (26.162, 21.971) ccw
  arc A55 (9.017, 26.035) -> (9.017, 25.273) centre (9.017, 25.654) ccw
  arc A56 (10.541, 27.813) -> (10.541, 28.575) centre (10.541, 28.194) ccw
  line L177 (27.686, 27.051) -> (26.162, 27.051)
  arc A57 (26.162, 22.352) -> (26.162, 21.59) centre (26.162, 21.971) ccw
  arc A58 (10.541, 32.893) -> (10.541, 33.655) centre (10.541, 33.274) ccw
  arc A59 (27.686, 34.29) -> (27.686, 35.052) centre (27.686, 34.671) ccw
  arc A60 (27.686, 24.13) -> (27.686, 24.892) centre (27.686, 24.511) ccw
  line L178 (10.541, 30.734) -> (9.017, 30.734)
  line L179 (27.686, 24.511) -> (26.162, 24.511)
  arc A61 (26.162, 35.052) -> (26.162, 34.29) centre (26.162, 34.671) ccw
  arc A62 (9.017, 31.115) -> (9.017, 30.353) centre (9.017, 30.734) ccw
  arc A63 (9.017, 26.035) -> (9.017, 25.273) centre (9.017, 25.654) ccw
  line L180 (10.541, 28.194) -> (9.017, 28.194)
  line L181 (27.686, 32.131) -> (26.162, 32.131)
  arc A64 (26.162, 29.972) -> (26.162, 29.21) centre (26.162, 29.591) ccw
  arc A65 (26.162, 27.432) -> (26.162, 26.67) centre (26.162, 27.051) ccw
  arc A66 (26.162, 24.892) -> (26.162, 24.13) centre (26.162, 24.511) ccw
  arc A67 (9.017, 28.575) -> (9.017, 27.813) centre (9.017, 28.194) ccw
  arc A68 (9.017, 28.575) -> (9.017, 27.813) centre (9.017, 28.194) ccw
  line L182 (27.686, 34.671) -> (26.162, 34.671)
  line L183 (27.686, 21.971) -> (26.162, 21.971)
  arc A69 (9.017, 33.655) -> (9.017, 32.893) centre (9.017, 33.274) ccw
  arc A70 (26.162, 37.592) -> (26.162, 36.83) centre (26.162, 37.211) ccw
  arc A71 (26.162, 32.512) -> (26.162, 31.75) centre (26.162, 32.131) ccw
  arc A72 (27.686, 29.21) -> (27.686, 29.972) centre (27.686, 29.591) ccw
  arc A73 (14.986, 26.67) -> (14.986, 27.432) centre (14.986, 27.051) ccw
  arc A74 (5.4846, 42.555) -> (4.5194, 42.555) centre (5.002, 42.555) ccw
  arc A75 (13.462, 32.512) -> (13.462, 31.75) centre (13.462, 32.131) ccw
  arc A76 (14.986, 34.29) -> (14.986, 35.052) centre (14.986, 34.671) ccw
  arc A77 (14.986, 31.75) -> (14.986, 32.512) centre (14.986, 32.131) ccw
  arc A78 (4.5194, 14.615) -> (5.4846, 14.615) centre (5.002, 14.615) ccw
  arc A79 (4.5194, 42.555) -> (5.4846, 42.555) centre (5.002, 42.555) ccw
  arc A80 (5.4846, 12.075) -> (4.5194, 12.075) centre (5.002, 12.075) ccw
  arc A81 (13.462, 37.592) -> (13.462, 36.83) centre (13.462, 37.211) ccw
  arc A82 (14.986, 29.21) -> (14.986, 29.972) centre (14.986, 29.591) ccw
  arc A83 (13.462, 24.892) -> (13.462, 24.13) centre (13.462, 24.511) ccw
  arc A84 (13.462, 29.972) -> (13.462, 29.21) centre (13.462, 29.591) ccw
  line L184 (13.462, 24.511) -> (14.986, 24.511)
  arc A85 (14.986, 29.21) -> (14.986, 29.972) centre (14.986, 29.591) ccw
  line L185 (13.462, 19.431) -> (14.986, 19.431)
  line L186 (13.462, 29.591) -> (14.986, 29.591)
  arc A86 (14.986, 31.75) -> (14.986, 32.512) centre (14.986, 32.131) ccw
  arc A87 (13.462, 22.352) -> (13.462, 21.59) centre (13.462, 21.971) ccw
  line L187 (13.462, 21.971) -> (14.986, 21.971)
  arc A88 (14.986, 21.59) -> (14.986, 22.352) centre (14.986, 21.971) ccw
  line L188 (13.462, 27.051) -> (14.986, 27.051)
  arc A89 (14.986, 24.13) -> (14.986, 24.892) centre (14.986, 24.511) ccw
  line L189 (13.462, 32.131) -> (14.986, 32.131)
  line L190 (13.462, 32.131) -> (14.986, 32.131)
  arc A90 (13.462, 27.432) -> (13.462, 26.67) centre (13.462, 27.051) ccw
  line L191 (13.462, 27.051) -> (14.986, 27.051)
  arc A91 (14.986, 21.59) -> (14.986, 22.352) centre (14.986, 21.971) ccw
  line L192 (13.462, 19.431) -> (14.986, 19.431)
  line L193 (27.686, 19.431) -> (26.162, 19.431)
  line L194 (13.462, 29.591) -> (14.986, 29.591)
  line L195 (27.686, 19.431) -> (26.162, 19.431)
  arc A92 (13.462, 24.892) -> (13.462, 24.13) centre (13.462, 24.511) ccw
  arc A93 (14.986, 24.13) -> (14.986, 24.892) centre (14.986, 24.511) ccw
  arc A94 (13.462, 27.432) -> (13.462, 26.67) centre (13.462, 27.051) ccw
  arc A95 (13.462, 19.812) -> (13.462, 19.05) centre (13.462, 19.431) ccw
  arc A96 (13.462, 35.052) -> (13.462, 34.29) centre (13.462, 34.671) ccw
  arc A97 (14.986, 26.67) -> (14.986, 27.432) centre (14.986, 27.051) ccw
  arc A98 (13.462, 37.592) -> (13.462, 36.83) centre (13.462, 37.211) ccw
  arc A99 (26.162, 19.812) -> (26.162, 19.05) centre (26.162, 19.431) ccw
  line L196 (13.462, 34.671) -> (14.986, 34.671)
  line L197 (13.462, 24.511) -> (14.986, 24.511)
  arc A100 (14.986, 19.05) -> (14.986, 19.812) centre (14.986, 19.431) ccw
  line L198 (13.462, 37.211) -> (14.986, 37.211)
  arc A101 (14.986, 36.83) -> (14.986, 37.592) centre (14.986, 37.211) ccw
  arc A102 (14.986, 34.29) -> (14.986, 35.052) centre (14.986, 34.671) ccw
  arc A103 (27.686, 19.05) -> (27.686, 19.812) centre (27.686, 19.431) ccw
  arc A104 (13.462, 22.352) -> (13.462, 21.59) centre (13.462, 21.971) ccw
  arc A105 (5.4846, 42.555) -> (4.5194, 42.555) centre (5.002, 42.555) ccw
  arc A106 (13.462, 35.052) -> (13.462, 34.29) centre (13.462, 34.671) ccw
  arc A107 (5.4846, 12.075) -> (4.5194, 12.075) centre (5.002, 12.075) ccw
  line L199 (13.462, 21.971) -> (14.986, 21.971)
  arc A108 (4.5194, 12.075) -> (5.4846, 12.075) centre (5.002, 12.075) ccw
  arc A109 (4.5194, 42.555) -> (5.4846, 42.555) centre (5.002, 42.555) ccw
  line L200 (13.462, 37.211) -> (14.986, 37.211)
  arc A110 (14.986, 19.05) -> (14.986, 19.812) centre (14.986, 19.431) ccw
  arc A111 (13.462, 19.812) -> (13.462, 19.05) centre (13.462, 19.431) ccw
  arc A112 (14.986, 36.83) -> (14.986, 37.592) centre (14.986, 37.211) ccw
  arc A113 (5.4846, 34.935) -> (4.5194, 34.935) centre (5.002, 34.935) ccw
  arc A114 (13.462, 29.972) -> (13.462, 29.21) centre (13.462, 29.591) ccw
  line L201 (13.462, 34.671) -> (14.986, 34.671)
  arc A115 (27.686, 21.59) -> (27.686, 22.352) centre (27.686, 21.971) ccw
  arc A116 (13.462, 32.512) -> (13.462, 31.75) centre (13.462, 32.131) ccw
  arc A117 (4.5194, 34.935) -> (5.4846, 34.935) centre (5.002, 34.935) ccw
  arc A118 (5.4846, 34.935) -> (4.5194, 34.935) centre (5.002, 34.935) ccw
  arc A119 (30.8896, 27.315) -> (29.9244, 27.315) centre (30.407, 27.315) ccw
  arc A120 (30.8896, 32.395) -> (29.9244, 32.395) centre (30.407, 32.395) ccw
  arc A121 (5.4846, 6.995) -> (4.5194, 6.995) centre (5.002, 6.995) ccw
  arc A122 (5.4846, 9.535) -> (4.5194, 9.535) centre (5.002, 9.535) ccw
  arc A123 (30.8896, 24.775) -> (29.9244, 24.775) centre (30.407, 24.775) ccw
  arc A124 (29.9244, 37.475) -> (30.8896, 37.475) centre (30.407, 37.475) ccw
  arc A125 (5.4846, 37.475) -> (4.5194, 37.475) centre (5.002, 37.475) ccw
  arc A126 (30.8896, 34.935) -> (29.9244, 34.935) centre (30.407, 34.935) ccw
  arc A127 (29.9244, 24.775) -> (30.8896, 24.775) centre (30.407, 24.775) ccw
  arc A128 (5.4846, 14.615) -> (4.5194, 14.615) centre (5.002, 14.615) ccw
  arc A129 (4.5194, 24.775) -> (5.4846, 24.775) centre (5.002, 24.775) ccw
  arc A130 (4.5194, 27.315) -> (5.4846, 27.315) centre (5.002, 27.315) ccw
  arc A131 (5.4846, 37.475) -> (4.5194, 37.475) centre (5.002, 37.475) ccw
  arc A132 (5.4846, 29.855) -> (4.5194, 29.855) centre (5.002, 29.855) ccw
  arc A133 (5.4846, 19.695) -> (4.5194, 19.695) centre (5.002, 19.695) ccw
  arc A134 (4.5194, 9.535) -> (5.4846, 9.535) centre (5.002, 9.535) ccw
  arc A135 (4.5194, 14.615) -> (5.4846, 14.615) centre (5.002, 14.615) ccw
  arc A136 (4.5194, 12.075) -> (5.4846, 12.075) centre (5.002, 12.075) ccw
  arc A137 (4.5194, 17.155) -> (5.4846, 17.155) centre (5.002, 17.155) ccw
  arc A138 (30.8896, 34.935) -> (29.9244, 34.935) centre (30.407, 34.935) ccw
  arc A139 (4.5194, 24.775) -> (5.4846, 24.775) centre (5.002, 24.775) ccw
  arc A140 (29.9244, 32.395) -> (30.8896, 32.395) centre (30.407, 32.395) ccw
  arc A141 (30.8896, 24.775) -> (29.9244, 24.775) centre (30.407, 24.775) ccw
  arc A142 (5.4846, 24.775) -> (4.5194, 24.775) centre (5.002, 24.775) ccw
  arc A143 (5.4846, 17.155) -> (4.5194, 17.155) centre (5.002, 17.155) ccw
  arc A144 (29.9244, 27.315) -> (30.8896, 27.315) centre (30.407, 27.315) ccw
  arc A145 (5.4846, 29.855) -> (4.5194, 29.855) centre (5.002, 29.855) ccw
  arc A146 (4.5194, 19.695) -> (5.4846, 19.695) centre (5.002, 19.695) ccw
  arc A147 (30.8896, 27.315) -> (29.9244, 27.315) centre (30.407, 27.315) ccw
  arc A148 (5.4846, 27.315) -> (4.5194, 27.315) centre (5.002, 27.315) ccw
  arc A149 (5.4846, 22.235) -> (4.5194, 22.235) centre (5.002, 22.235) ccw
  arc A150 (5.4846, 27.315) -> (4.5194, 27.315) centre (5.002, 27.315) ccw
  arc A151 (4.5194, 6.995) -> (5.4846, 6.995) centre (5.002, 6.995) ccw
  arc A152 (5.4846, 24.775) -> (4.5194, 24.775) centre (5.002, 24.775) ccw
  arc A153 (4.5194, 37.475) -> (5.4846, 37.475) centre (5.002, 37.475) ccw
  arc A154 (29.9244, 29.855) -> (30.8896, 29.855) centre (30.407, 29.855) ccw
  arc A155 (4.5194, 34.935) -> (5.4846, 34.935) centre (5.002, 34.935) ccw
  arc A156 (29.9244, 34.935) -> (30.8896, 34.935) centre (30.407, 34.935) ccw
  arc A157 (5.4846, 19.695) -> (4.5194, 19.695) centre (5.002, 19.695) ccw
  arc A158 (5.4846, 6.995) -> (4.5194, 6.995) centre (5.002, 6.995) ccw
  arc A159 (4.5194, 9.535) -> (5.4846, 9.535) centre (5.002, 9.535) ccw
  arc A160 (5.4846, 14.615) -> (4.5194, 14.615) centre (5.002, 14.615) ccw
  arc A161 (4.5194, 17.155) -> (5.4846, 17.155) centre (5.002, 17.155) ccw
  arc A162 (5.4846, 17.155) -> (4.5194, 17.155) centre (5.002, 17.155) ccw
  arc A163 (5.4846, 32.395) -> (4.5194, 32.395) centre (5.002, 32.395) ccw
  arc A164 (5.4846, 32.395) -> (4.5194, 32.395) centre (5.002, 32.395) ccw
  arc A165 (29.9244, 24.775) -> (30.8896, 24.775) centre (30.407, 24.775) ccw
  arc A166 (29.9244, 34.935) -> (30.8896, 34.935) centre (30.407, 34.935) ccw
  arc A167 (4.5194, 29.855) -> (5.4846, 29.855) centre (5.002, 29.855) ccw
  arc A168 (5.4846, 9.535) -> (4.5194, 9.535) centre (5.002, 9.535) ccw
  arc A169 (30.8896, 32.395) -> (29.9244, 32.395) centre (30.407, 32.395) ccw
  arc A170 (4.5194, 22.235) -> (5.4846, 22.235) centre (5.002, 22.235) ccw
  arc A171 (4.5194, 19.695) -> (5.4846, 19.695) centre (5.002, 19.695) ccw
  arc A172 (4.5194, 37.475) -> (5.4846, 37.475) centre (5.002, 37.475) ccw
  arc A173 (4.5194, 6.995) -> (5.4846, 6.995) centre (5.002, 6.995) ccw
  arc A174 (4.5194, 32.395) -> (5.4846, 32.395) centre (5.002, 32.395) ccw
  arc A175 (4.5194, 22.235) -> (5.4846, 22.235) centre (5.002, 22.235) ccw
  arc A176 (30.8896, 37.475) -> (29.9244, 37.475) centre (30.407, 37.475) ccw
  arc A177 (5.4846, 22.235) -> (4.5194, 22.235) centre (5.002, 22.235) ccw
  arc A178 (4.5194, 27.315) -> (5.4846, 27.315) centre (5.002, 27.315) ccw
  arc A179 (29.9244, 32.395) -> (30.8896, 32.395) centre (30.407, 32.395) ccw
  arc A180 (4.5194, 32.395) -> (5.4846, 32.395) centre (5.002, 32.395) ccw
  arc A181 (29.9244, 37.475) -> (30.8896, 37.475) centre (30.407, 37.475) ccw
  arc A182 (29.9244, 27.315) -> (30.8896, 27.315) centre (30.407, 27.315) ccw
  arc A183 (5.4846, 40.015) -> (4.5194, 40.015) centre (5.002, 40.015) ccw
  arc A184 (30.8896, 12.075) -> (29.9244, 12.075) centre (30.407, 12.075) ccw
  arc A185 (5.4846, 40.015) -> (4.5194, 40.015) centre (5.002, 40.015) ccw
  arc A186 (30.8896, 22.235) -> (29.9244, 22.235) centre (30.407, 22.235) ccw
  arc A187 (4.5194, 40.015) -> (5.4846, 40.015) centre (5.002, 40.015) ccw
  arc A188 (29.9244, 12.075) -> (30.8896, 12.075) centre (30.407, 12.075) ccw
  arc A189 (4.5194, 40.015) -> (5.4846, 40.015) centre (5.002, 40.015) ccw
  arc A190 (30.8896, 14.615) -> (29.9244, 14.615) centre (30.407, 14.615) ccw
  arc A191 (30.8896, 14.615) -> (29.9244, 14.615) centre (30.407, 14.615) ccw
  arc A192 (29.9244, 42.555) -> (30.8896, 42.555) centre (30.407, 42.555) ccw
  arc A193 (29.9244, 29.855) -> (30.8896, 29.855) centre (30.407, 29.855) ccw
  arc A194 (29.9244, 22.235) -> (30.8896, 22.235) centre (30.407, 22.235) ccw
  arc A195 (30.8896, 6.995) -> (29.9244, 6.995) centre (30.407, 6.995) ccw
  arc A196 (30.8896, 6.995) -> (29.9244, 6.995) centre (30.407, 6.995) ccw
  arc A197 (30.8896, 19.695) -> (29.9244, 19.695) centre (30.407, 19.695) ccw
  arc A198 (30.8896, 22.235) -> (29.9244, 22.235) centre (30.407, 22.235) ccw
  arc A199 (30.8896, 17.155) -> (29.9244, 17.155) centre (30.407, 17.155) ccw
  arc A200 (29.9244, 9.535) -> (30.8896, 9.535) centre (30.407, 9.535) ccw
  arc A201 (29.9244, 17.155) -> (30.8896, 17.155) centre (30.407, 17.155) ccw
  arc A202 (30.8896, 9.535) -> (29.9244, 9.535) centre (30.407, 9.535) ccw
  arc A203 (29.9244, 17.155) -> (30.8896, 17.155) centre (30.407, 17.155) ccw
  arc A204 (30.8896, 40.015) -> (29.9244, 40.015) centre (30.407, 40.015) ccw
  arc A205 (30.8896, 40.015) -> (29.9244, 40.015) centre (30.407, 40.015) ccw
  arc A206 (29.9244, 14.615) -> (30.8896, 14.615) centre (30.407, 14.615) ccw
  arc A207 (30.8896, 9.535) -> (29.9244, 9.535) centre (30.407, 9.535) ccw
  arc A208 (29.9244, 40.015) -> (30.8896, 40.015) centre (30.407, 40.015) ccw
  arc A209 (30.8896, 42.555) -> (29.9244, 42.555) centre (30.407, 42.555) ccw
  arc A210 (29.9244, 6.995) -> (30.8896, 6.995) centre (30.407, 6.995) ccw
  arc A211 (30.8896, 37.475) -> (29.9244, 37.475) centre (30.407, 37.475) ccw
  arc A212 (29.9244, 19.695) -> (30.8896, 19.695) centre (30.407, 19.695) ccw
  arc A213 (29.9244, 42.555) -> (30.8896, 42.555) centre (30.407, 42.555) ccw
  arc A214 (30.8896, 29.855) -> (29.9244, 29.855) centre (30.407, 29.855) ccw
  arc A215 (29.9244, 40.015) -> (30.8896, 40.015) centre (30.407, 40.015) ccw
  arc A216 (30.8896, 17.155) -> (29.9244, 17.155) centre (30.407, 17.155) ccw
  arc A217 (30.8896, 19.695) -> (29.9244, 19.695) centre (30.407, 19.695) ccw
  arc A218 (29.9244, 12.075) -> (30.8896, 12.075) centre (30.407, 12.075) ccw
  arc A219 (29.9244, 9.535) -> (30.8896, 9.535) centre (30.407, 9.535) ccw
  arc A220 (29.9244, 19.695) -> (30.8896, 19.695) centre (30.407, 19.695) ccw
  arc A221 (4.5194, 29.855) -> (5.4846, 29.855) centre (5.002, 29.855) ccw
  arc A222 (30.8896, 42.555) -> (29.9244, 42.555) centre (30.407, 42.555) ccw
  arc A223 (30.8896, 12.075) -> (29.9244, 12.075) centre (30.407, 12.075) ccw
  arc A224 (30.8896, 29.855) -> (29.9244, 29.855) centre (30.407, 29.855) ccw
  arc A225 (29.9244, 14.615) -> (30.8896, 14.615) centre (30.407, 14.615) ccw